Autodesk Fusion 360 part; units mm, degrees
note: some values were not read from the file. Chosen so that the rebuilt part matches the saved one: which face or edge a step refers to. Set by a fixed rule: which sketch regions a step uses.
(part 2 of 3)
  line L673 (81.1779, -7.0016) -> (84.5538, -8.9507)
  line L674 (81.1779, -3.1036) -> (81.1779, -7.0016)
  line L675 (84.5538, -1.1545) -> (81.1779, -3.1036)
  line L676 (87.9296, -3.1036) -> (84.5538, -1.1545)
  line L677 (84.5538, -8.9507) -> (87.9296, -7.0016)
  line L678 (83.9508, -13.893) -> (83.9508, -9.995)
  line L679 (83.9508, -9.995) -> (80.575, -8.0459)
  line L680 (80.575, -8.0459) -> (77.1992, -9.995)
  line L681 (77.1992, -9.995) -> (77.1992, -13.893)
  line L682 (77.1992, -13.893) -> (80.575, -15.8421)
  line L683 (80.575, -15.8421) -> (83.9508, -13.893)
  line L684 (87.9296, -7.0016) -> (87.9296, -3.1036)
  line L685 (9.5604, 6.9424) -> (12.9363, 4.9933)
  line L686 (9.5604, 10.8404) -> (9.5604, 6.9424)
  line L687 (12.9363, 12.7895) -> (9.5604, 10.8404)
  line L688 (16.3121, 10.8404) -> (12.9363, 12.7895)
  line L689 (12.9363, 4.9933) -> (16.3121, 6.9424)
  line L690 (12.3333, 0.051) -> (12.3333, 3.949)
  line L691 (12.3333, 3.949) -> (8.9575, 5.8981)
  line L692 (8.9575, 5.8981) -> (5.5817, 3.949)
  line L693 (5.5817, 3.949) -> (5.5817, 0.051)
  line L694 (5.5817, 0.051) -> (8.9575, -1.8981)
  line L695 (8.9575, -1.8981) -> (12.3333, 0.051)
  line L696 (16.3121, 6.9424) -> (16.3121, 10.8404)
  line L697 (17.5179, 6.9424) -> (20.8938, 4.9933)
  line L698 (17.5179, 10.8404) -> (17.5179, 6.9424)
  line L699 (20.8938, 12.7895) -> (17.5179, 10.8404)
  line L700 (24.2696, 10.8404) -> (20.8938, 12.7895)
  line L701 (20.8938, 4.9933) -> (24.2696, 6.9424)
  line L702 (20.2908, 0.051) -> (20.2908, 3.949)
  line L703 (20.2908, 3.949) -> (16.915, 5.8981)
  line L704 (16.915, 5.8981) -> (13.5392, 3.949)
  line L705 (13.5392, 3.949) -> (13.5392, 0.051)
  line L706 (13.5392, 0.051) -> (16.915, -1.8981)
  line L707 (16.915, -1.8981) -> (20.2908, 0.051)
  line L708 (24.2696, 6.9424) -> (24.2696, 10.8404)
  line L709 (25.4754, 6.9424) -> (28.8513, 4.9933)
  line L710 (25.4754, 10.8404) -> (25.4754, 6.9424)
  line L711 (28.8513, 12.7895) -> (25.4754, 10.8404)
  line L712 (32.2271, 10.8404) -> (28.8513, 12.7895)
  line L713 (28.8513, 4.9933) -> (32.2271, 6.9424)
  line L714 (28.2483, 0.051) -> (28.2483, 3.949)
  line L715 (28.2483, 3.949) -> (24.8725, 5.8981)
  line L716 (24.8725, 5.8981) -> (21.4967, 3.949)
  line L717 (21.4967, 3.949) -> (21.4967, 0.051)
  line L718 (21.4967, 0.051) -> (24.8725, -1.8981)
  line L719 (24.8725, -1.8981) -> (28.2483, 0.051)
  line L720 (32.2271, 6.9424) -> (32.2271, 10.8404)
  line L721 (33.4329, 6.9424) -> (36.8088, 4.9933)
  line L722 (33.4329, 10.8404) -> (33.4329, 6.9424)
  line L723 (36.8088, 12.7895) -> (33.4329, 10.8404)
  line L724 (40.1846, 10.8404) -> (36.8088, 12.7895)
  line L725 (36.8088, 4.9933) -> (40.1846, 6.9424)
  line L726 (36.2058, 0.051) -> (36.2058, 3.949)
  line L727 (36.2058, 3.949) -> (32.83, 5.8981)
  line L728 (32.83, 5.8981) -> (29.4542, 3.949)
  line L729 (29.4542, 3.949) -> (29.4542, 0.051)
  line L730 (29.4542, 0.051) -> (32.83, -1.8981)
  line L731 (32.83, -1.8981) -> (36.2058, 0.051)
  line L732 (40.1846, 6.9424) -> (40.1846, 10.8404)
  line L733 (41.3904, 6.9424) -> (44.7663, 4.9933)
  line L734 (41.3904, 10.8404) -> (41.3904, 6.9424)
  line L735 (44.7663, 12.7895) -> (41.3904, 10.8404)
  line L736 (48.1421, 10.8404) -> (44.7663, 12.7895)
  line L737 (44.7663, 4.9933) -> (48.1421, 6.9424)
  line L738 (44.1633, 0.051) -> (44.1633, 3.949)
  line L739 (44.1633, 3.949) -> (40.7875, 5.8981)
  line L740 (40.7875, 5.8981) -> (37.4117, 3.949)
  line L741 (37.4117, 3.949) -> (37.4117, 0.051)
  line L742 (37.4117, 0.051) -> (40.7875, -1.8981)
  line L743 (40.7875, -1.8981) -> (44.1633, 0.051)
  line L744 (48.1421, 6.9424) -> (48.1421, 10.8404)
  line L745 (49.3479, 6.9424) -> (52.7238, 4.9933)
  line L746 (49.3479, 10.8404) -> (49.3479, 6.9424)
  line L747 (52.7238, 12.7895) -> (49.3479, 10.8404)
  line L748 (56.0996, 10.8404) -> (52.7238, 12.7895)
  line L749 (52.7238, 4.9933) -> (56.0996, 6.9424)
  line L750 (52.1208, 0.051) -> (52.1208, 3.949)
  line L751 (52.1208, 3.949) -> (48.745, 5.8981)
  line L752 (48.745, 5.8981) -> (45.3692, 3.949)
  line L753 (45.3692, 3.949) -> (45.3692, 0.051)
  line L754 (45.3692, 0.051) -> (48.745, -1.8981)
  line L755 (48.745, -1.8981) -> (52.1208, 0.051)
  line L756 (56.0996, 6.9424) -> (56.0996, 10.8404)
  line L757 (57.3054, 6.9424) -> (60.6813, 4.9933)
  line L758 (57.3054, 10.8404) -> (57.3054, 6.9424)
  line L759 (60.6813, 12.7895) -> (57.3054, 10.8404)
  line L760 (64.0571, 10.8404) -> (60.6813, 12.7895)
  line L761 (60.6813, 4.9933) -> (64.0571, 6.9424)
  line L762 (60.0783, 0.051) -> (60.0783, 3.949)
  line L763 (60.0783, 3.949) -> (56.7025, 5.8981)
  line L764 (56.7025, 5.8981) -> (53.3267, 3.949)
  line L765 (53.3267, 3.949) -> (53.3267, 0.051)
  line L766 (53.3267, 0.051) -> (56.7025, -1.8981)
  line L767 (56.7025, -1.8981) -> (60.0783, 0.051)
  line L768 (64.0571, 6.9424) -> (64.0571, 10.8404)
  line L769 (65.2629, 6.9424) -> (68.6388, 4.9933)
  line L770 (65.2629, 10.8404) -> (65.2629, 6.9424)
  line L771 (68.6388, 12.7895) -> (65.2629, 10.8404)
  line L772 (72.0146, 10.8404) -> (68.6388, 12.7895)
  line L773 (68.6388, 4.9933) -> (72.0146, 6.9424)
  line L774 (68.0358, 0.051) -> (68.0358, 3.949)
  line L775 (68.0358, 3.949) -> (64.66, 5.8981)
  line L776 (64.66, 5.8981) -> (61.2842, 3.949)
  line L777 (61.2842, 3.949) -> (61.2842, 0.051)
  line L778 (61.2842, 0.051) -> (64.66, -1.8981)
  line L779 (64.66, -1.8981) -> (68.0358, 0.051)
  line L780 (72.0146, 6.9424) -> (72.0146, 10.8404)
  line L781 (73.2204, 6.9424) -> (76.5963, 4.9933)
  line L782 (73.2204, 10.8404) -> (73.2204, 6.9424)
  line L783 (76.5963, 12.7895) -> (73.2204, 10.8404)
  line L784 (79.9721, 10.8404) -> (76.5963, 12.7895)
  line L785 (76.5963, 4.9933) -> (79.9721, 6.9424)
  line L786 (75.9933, 0.051) -> (75.9933, 3.949)
  line L787 (75.9933, 3.949) -> (72.6175, 5.8981)
  line L788 (72.6175, 5.8981) -> (69.2417, 3.949)
  line L789 (69.2417, 3.949) -> (69.2417, 0.051)
  line L790 (69.2417, 0.051) -> (72.6175, -1.8981)
  line L791 (72.6175, -1.8981) -> (75.9933, 0.051)
  line L792 (79.9721, 6.9424) -> (79.9721, 10.8404)
  line L793 (81.1779, 6.9424) -> (84.5538, 4.9933)
  line L794 (81.1779, 10.8404) -> (81.1779, 6.9424)
  line L795 (84.5538, 12.7895) -> (81.1779, 10.8404)
  line L796 (87.9296, 10.8404) -> (84.5538, 12.7895)
  line L797 (84.5538, 4.9933) -> (87.9296, 6.9424)
  line L798 (83.9508, 0.051) -> (83.9508, 3.949)
  line L799 (83.9508, 3.949) -> (80.575, 5.8981)
  line L800 (80.575, 5.8981) -> (77.1992, 3.949)
  line L801 (77.1992, 3.949) -> (77.1992, 0.051)
  line L802 (77.1992, 0.051) -> (80.575, -1.8981)
  line L803 (80.575, -1.8981) -> (83.9508, 0.051)
  line L804 (87.9296, 6.9424) -> (87.9296, 10.8404)
  line L805 (1.6029, 20.8864) -> (4.9788, 18.9373)
  line L806 (1.6029, 24.7844) -> (1.6029, 20.8864)
  line L807 (4.9788, 26.7335) -> (1.6029, 24.7844)
  line L808 (8.3546, 24.7844) -> (4.9788, 26.7335)
  line L809 (4.9788, 18.9373) -> (8.3546, 20.8864)
  line L810 (4.3758, 13.995) -> (4.3758, 17.893)
  line L811 (4.3758, 17.893) -> (1, 19.8421)
  line L812 (1, 19.8421) -> (-2.3758, 17.893)
  line L813 (-2.3758, 17.893) -> (-2.3758, 13.995)
  line L814 (-2.3758, 13.995) -> (1, 12.0459)
  line L815 (1, 12.0459) -> (4.3758, 13.995)
  line L816 (8.3546, 20.8864) -> (8.3546, 24.7844)
  line L817 (9.5604, 20.8864) -> (12.9363, 18.9373)
  line L818 (9.5604, 24.7844) -> (9.5604, 20.8864)
  line L819 (12.9363, 26.7335) -> (9.5604, 24.7844)
  line L820 (16.3121, 24.7844) -> (12.9363, 26.7335)
  line L821 (12.9363, 18.9373) -> (16.3121, 20.8864)
  line L822 (12.3333, 13.995) -> (12.3333, 17.893)
  line L823 (12.3333, 17.893) -> (8.9575, 19.8421)
  line L824 (8.9575, 19.8421) -> (5.5817, 17.893)
  line L825 (5.5817, 17.893) -> (5.5817, 13.995)
  line L826 (5.5817, 13.995) -> (8.9575, 12.0459)
  line L827 (8.9575, 12.0459) -> (12.3333, 13.995)
  line L828 (16.3121, 20.8864) -> (16.3121, 24.7844)
  line L829 (17.5179, 20.8864) -> (20.8938, 18.9373)
  line L830 (17.5179, 24.7844) -> (17.5179, 20.8864)
  line L831 (20.8938, 26.7335) -> (17.5179, 24.7844)
  line L832 (24.2696, 24.7844) -> (20.8938, 26.7335)
  line L833 (20.8938, 18.9373) -> (24.2696, 20.8864)
  line L834 (20.2908, 13.995) -> (20.2908, 17.893)
  line L835 (20.2908, 17.893) -> (16.915, 19.8421)
  line L836 (16.915, 19.8421) -> (13.5392, 17.893)
  line L837 (13.5392, 17.893) -> (13.5392, 13.995)
  line L838 (13.5392, 13.995) -> (16.915, 12.0459)
  line L839 (16.915, 12.0459) -> (20.2908, 13.995)
  line L840 (24.2696, 20.8864) -> (24.2696, 24.7844)
  line L841 (25.4754, 20.8864) -> (28.8513, 18.9373)
  line L842 (25.4754, 24.7844) -> (25.4754, 20.8864)
  line L843 (28.8513, 26.7335) -> (25.4754, 24.7844)
  line L844 (32.2271, 24.7844) -> (28.8513, 26.7335)
  line L845 (28.8513, 18.9373) -> (32.2271, 20.8864)
  line L846 (28.2483, 13.995) -> (28.2483, 17.893)
  line L847 (28.2483, 17.893) -> (24.8725, 19.8421)
  line L848 (24.8725, 19.8421) -> (21.4967, 17.893)
  line L849 (21.4967, 17.893) -> (21.4967, 13.995)
  line L850 (21.4967, 13.995) -> (24.8725, 12.0459)
  line L851 (24.8725, 12.0459) -> (28.2483, 13.995)
  line L852 (32.2271, 20.8864) -> (32.2271, 24.7844)
  line L853 (33.4329, 20.8864) -> (36.8088, 18.9373)
  line L854 (33.4329, 24.7844) -> (33.4329, 20.8864)
  line L855 (36.8088, 26.7335) -> (33.4329, 24.7844)
  line L856 (40.1846, 24.7844) -> (36.8088, 26.7335)
  line L857 (36.8088, 18.9373) -> (40.1846, 20.8864)
  line L858 (36.2058, 13.995) -> (36.2058, 17.893)
  line L859 (36.2058, 17.893) -> (32.83, 19.8421)
  line L860 (32.83, 19.8421) -> (29.4542, 17.893)
  line L861 (29.4542, 17.893) -> (29.4542, 13.995)
  line L862 (29.4542, 13.995) -> (32.83, 12.0459)
  line L863 (32.83, 12.0459) -> (36.2058, 13.995)
  line L864 (40.1846, 20.8864) -> (40.1846, 24.7844)
  line L865 (41.3904, 20.8864) -> (44.7663, 18.9373)
  line L866 (41.3904, 24.7844) -> (41.3904, 20.8864)
  line L867 (44.7663, 26.7335) -> (41.3904, 24.7844)
  line L868 (48.1421, 24.7844) -> (44.7663, 26.7335)
  line L869 (44.7663, 18.9373) -> (48.1421, 20.8864)
  line L870 (44.1633, 13.995) -> (44.1633, 17.893)
  line L871 (44.1633, 17.893) -> (40.7875, 19.8421)
  line L872 (40.7875, 19.8421) -> (37.4117, 17.893)
  line L873 (37.4117, 17.893) -> (37.4117, 13.995)
  line L874 (37.4117, 13.995) -> (40.7875, 12.0459)
  line L875 (40.7875, 12.0459) -> (44.1633, 13.995)
  line L876 (48.1421, 20.8864) -> (48.1421, 24.7844)
  line L877 (49.3479, 20.8864) -> (52.7238, 18.9373)
  line L878 (49.3479, 24.7844) -> (49.3479, 20.8864)
  line L879 (52.7238, 26.7335) -> (49.3479, 24.7844)
  line L880 (56.0996, 24.7844) -> (52.7238, 26.7335)
  line L881 (52.7238, 18.9373) -> (56.0996, 20.8864)
  line L882 (52.1208, 13.995) -> (52.1208, 17.893)
  line L883 (52.1208, 17.893) -> (48.745, 19.8421)
  line L884 (48.745, 19.8421) -> (45.3692, 17.893)
  line L885 (45.3692, 17.893) -> (45.3692, 13.995)
  line L886 (45.3692, 13.995) -> (48.745, 12.0459)
  line L887 (48.745, 12.0459) -> (52.1208, 13.995)
  line L888 (56.0996, 20.8864) -> (56.0996, 24.7844)
  line L889 (57.3054, 20.8864) -> (60.6813, 18.9373)
  line L890 (57.3054, 24.7844) -> (57.3054, 20.8864)
  line L891 (60.6813, 26.7335) -> (57.3054, 24.7844)
  line L892 (64.0571, 24.7844) -> (60.6813, 26.7335)
  line L893 (60.6813, 18.9373) -> (64.0571, 20.8864)
  line L894 (60.0783, 13.995) -> (60.0783, 17.893)
  line L895 (60.0783, 17.893) -> (56.7025, 19.8421)
  line L896 (56.7025, 19.8421) -> (53.3267, 17.893)
  line L897 (53.3267, 17.893) -> (53.3267, 13.995)
  line L898 (53.3267, 13.995) -> (56.7025, 12.0459)
  line L899 (56.7025, 12.0459) -> (60.0783, 13.995)
  line L900 (64.0571, 20.8864) -> (64.0571, 24.7844)
  line L901 (65.2629, 20.8864) -> (68.6388, 18.9373)
  line L902 (65.2629, 24.7844) -> (65.2629, 20.8864)
  line L903 (68.6388, 26.7335) -> (65.2629, 24.7844)
  line L904 (72.0146, 24.7844) -> (68.6388, 26.7335)
  line L905 (68.6388, 18.9373) -> (72.0146, 20.8864)
  line L906 (68.0358, 13.995) -> (68.0358, 17.893)
  line L907 (68.0358, 17.893) -> (64.66, 19.8421)
  line L908 (64.66, 19.8421) -> (61.2842, 17.893)
  line L909 (61.2842, 17.893) -> (61.2842, 13.995)
  line L910 (61.2842, 13.995) -> (64.66, 12.0459)
  line L911 (64.66, 12.0459) -> (68.0358, 13.995)
  line L912 (72.0146, 20.8864) -> (72.0146, 24.7844)
  line L913 (73.2204, 20.8864) -> (76.5963, 18.9373)
  line L914 (73.2204, 24.7844) -> (73.2204, 20.8864)
  line L915 (76.5963, 26.7335) -> (73.2204, 24.7844)
  line L916 (79.9721, 24.7844) -> (76.5963, 26.7335)
  line L917 (76.5963, 18.9373) -> (79.9721, 20.8864)
  line L918 (75.9933, 13.995) -> (75.9933, 17.893)
  line L919 (75.9933, 17.893) -> (72.6175, 19.8421)
  line L920 (72.6175, 19.8421) -> (69.2417, 17.893)
  line L921 (69.2417, 17.893) -> (69.2417, 13.995)
  line L922 (69.2417, 13.995) -> (72.6175, 12.0459)
  line L923 (72.6175, 12.0459) -> (75.9933, 13.995)
  line L924 (79.9721, 20.8864) -> (79.9721, 24.7844)
  line L925 (81.1779, 20.8864) -> (84.5538, 18.9373)
  line L926 (81.1779, 24.7844) -> (81.1779, 20.8864)
  line L927 (84.5538, 26.7335) -> (81.1779, 24.7844)
  line L928 (87.9296, 24.7844) -> (84.5538, 26.7335)
  line L929 (84.5538, 18.9373) -> (87.9296, 20.8864)
  line L930 (83.9508, 13.995) -> (83.9508, 17.893)
  line L931 (83.9508, 17.893) -> (80.575, 19.8421)
  line L932 (80.575, 19.8421) -> (77.1992, 17.893)
  line L933 (77.1992, 17.893) -> (77.1992, 13.995)
  line L934 (77.1992, 13.995) -> (80.575, 12.0459)
  line L935 (80.575, 12.0459) -> (83.9508, 13.995)
  line L936 (87.9296, 20.8864) -> (87.9296, 24.7844)
  line L937 (1.6029, 34.8304) -> (4.9788, 32.8813)
  line L938 (1.6029, 38.7284) -> (1.6029, 34.8304)
  line L939 (4.9788, 40.6775) -> (1.6029, 38.7284)
  line L940 (8.3546, 38.7284) -> (4.9788, 40.6775)
  line L941 (4.9788, 32.8813) -> (8.3546, 34.8304)
  line L942 (4.3758, 27.939) -> (4.3758, 31.837)
  line L943 (4.3758, 31.837) -> (1, 33.7861)
  line L944 (1, 33.7861) -> (-2.3758, 31.837)
  line L945 (-2.3758, 31.837) -> (-2.3758, 27.939)
  line L946 (-2.3758, 27.939) -> (1, 25.9899)
  line L947 (1, 25.9899) -> (4.3758, 27.939)
  line L948 (8.3546, 34.8304) -> (8.3546, 38.7284)
  line L949 (9.5604, 34.8304) -> (12.9363, 32.8813)
  line L950 (9.5604, 38.7284) -> (9.5604, 34.8304)
  line L951 (12.9363, 40.6775) -> (9.5604, 38.7284)
  line L952 (16.3121, 38.7284) -> (12.9363, 40.6775)
  line L953 (12.9363, 32.8813) -> (16.3121, 34.8304)
  line L954 (12.3333, 27.939) -> (12.3333, 31.837)
  line L955 (12.3333, 31.837) -> (8.9575, 33.7861)
  line L956 (8.9575, 33.7861) -> (5.5817, 31.837)
  line L957 (5.5817, 31.837) -> (5.5817, 27.939)
  line L958 (5.5817, 27.939) -> (8.9575, 25.9899)
  line L959 (8.9575, 25.9899) -> (12.3333, 27.939)
  line L960 (16.3121, 34.8304) -> (16.3121, 38.7284)
  line L961 (17.5179, 34.8304) -> (20.8938, 32.8813)
  line L962 (17.5179, 38.7284) -> (17.5179, 34.8304)
  line L963 (20.8938, 40.6775) -> (17.5179, 38.7284)
  line L964 (24.2696, 38.7284) -> (20.8938, 40.6775)
  line L965 (20.8938, 32.8813) -> (24.2696, 34.8304)
  line L966 (20.2908, 27.939) -> (20.2908, 31.837)
  line L967 (20.2908, 31.837) -> (16.915, 33.7861)
  line L968 (16.915, 33.7861) -> (13.5392, 31.837)
  line L969 (13.5392, 31.837) -> (13.5392, 27.939)
  line L970 (13.5392, 27.939) -> (16.915, 25.9899)
  line L971 (16.915, 25.9899) -> (20.2908, 27.939)
  line L972 (24.2696, 34.8304) -> (24.2696, 38.7284)
  line L973 (25.4754, 34.8304) -> (28.8513, 32.8813)
  line L974 (25.4754, 38.7284) -> (25.4754, 34.8304)
  line L975 (28.8513, 40.6775) -> (25.4754, 38.7284)
  line L976 (32.2271, 38.7284) -> (28.8513, 40.6775)
  line L977 (28.8513, 32.8813) -> (32.2271, 34.8304)
  line L978 (28.2483, 27.939) -> (28.2483, 31.837)
  line L979 (28.2483, 31.837) -> (24.8725, 33.7861)
  line L980 (24.8725, 33.7861) -> (21.4967, 31.837)
  line L981 (21.4967, 31.837) -> (21.4967, 27.939)
  line L982 (21.4967, 27.939) -> (24.8725, 25.9899)
  line L983 (24.8725, 25.9899) -> (28.2483, 27.939)
  line L984 (32.2271, 34.8304) -> (32.2271, 38.7284)
  line L985 (33.4329, 34.8304) -> (36.8088, 32.8813)
  line L986 (33.4329, 38.7284) -> (33.4329, 34.8304)
  line L987 (36.8088, 40.6775) -> (33.4329, 38.7284)
  line L988 (40.1846, 38.7284) -> (36.8088, 40.6775)
  line L989 (36.8088, 32.8813) -> (40.1846, 34.8304)
  line L990 (36.2058, 27.939) -> (36.2058, 31.837)
  line L991 (36.2058, 31.837) -> (32.83, 33.7861)
  line L992 (32.83, 33.7861) -> (29.4542, 31.837)
  line L993 (29.4542, 31.837) -> (29.4542, 27.939)
  line L994 (29.4542, 27.939) -> (32.83, 25.9899)
  line L995 (32.83, 25.9899) -> (36.2058, 27.939)
  line L996 (40.1846, 34.8304) -> (40.1846, 38.7284)
  line L997 (41.3904, 34.8304) -> (44.7663, 32.8813)
  line L998 (41.3904, 38.7284) -> (41.3904, 34.8304)
  line L999 (44.7663, 40.6775) -> (41.3904, 38.7284)
  line L1000 (48.1421, 38.7284) -> (44.7663, 40.6775)
  line L1001 (44.7663, 32.8813) -> (48.1421, 34.8304)
  line L1002 (44.1633, 27.939) -> (44.1633, 31.837)
  line L1003 (44.1633, 31.837) -> (40.7875, 33.7861)
  line L1004 (40.7875, 33.7861) -> (37.4117, 31.837)
  line L1005 (37.4117, 31.837) -> (37.4117, 27.939)
  line L1006 (37.4117, 27.939) -> (40.7875, 25.9899)
  line L1007 (40.7875, 25.9899) -> (44.1633, 27.939)
  line L1008 (48.1421, 34.8304) -> (48.1421, 38.7284)
  line L1009 (49.3479, 34.8304) -> (52.7238, 32.8813)
  line L1010 (49.3479, 38.7284) -> (49.3479, 34.8304)
  line L1011 (52.7238, 40.6775) -> (49.3479, 38.7284)
  line L1012 (56.0996, 38.7284) -> (52.7238, 40.6775)
  line L1013 (52.7238, 32.8813) -> (56.0996, 34.8304)
  line L1014 (52.1208, 27.939) -> (52.1208, 31.837)
  line L1015 (52.1208, 31.837) -> (48.745, 33.7861)
  line L1016 (48.745, 33.7861) -> (45.3692, 31.837)
  line L1017 (45.3692, 31.837) -> (45.3692, 27.939)
  line L1018 (45.3692, 27.939) -> (48.745, 25.9899)
  line L1019 (48.745, 25.9899) -> (52.1208, 27.939)
  line L1020 (56.0996, 34.8304) -> (56.0996, 38.7284)
  line L1021 (57.3054, 34.8304) -> (60.6813, 32.8813)
  line L1022 (57.3054, 38.7284) -> (57.3054, 34.8304)
  line L1023 (60.6813, 40.6775) -> (57.3054, 38.7284)
  line L1024 (64.0571, 38.7284) -> (60.6813, 40.6775)
  line L1025 (60.6813, 32.8813) -> (64.0571, 34.8304)
  line L1026 (60.0783, 27.939) -> (60.0783, 31.837)
  line L1027 (60.0783, 31.837) -> (56.7025, 33.7861)
  line L1028 (56.7025, 33.7861) -> (53.3267, 31.837)
  line L1029 (53.3267, 31.837) -> (53.3267, 27.939)
  line L1030 (53.3267, 27.939) -> (56.7025, 25.9899)
  line L1031 (56.7025, 25.9899) -> (60.0783, 27.939)
  line L1032 (64.0571, 34.8304) -> (64.0571, 38.7284)
  line L1033 (65.2629, 34.8304) -> (68.6388, 32.8813)
  line L1034 (65.2629, 38.7284) -> (65.2629, 34.8304)
  line L1035 (68.6388, 40.6775) -> (65.2629, 38.7284)
  line L1036 (72.0146, 38.7284) -> (68.6388, 40.6775)
  line L1037 (68.6388, 32.8813) -> (72.0146, 34.8304)
  line L1038 (68.0358, 27.939) -> (68.0358, 31.837)
  line L1039 (68.0358, 31.837) -> (64.66, 33.7861)
  line L1040 (64.66, 33.7861) -> (61.2842, 31.837)
  line L1041 (61.2842, 31.837) -> (61.2842, 27.939)
  line L1042 (61.2842, 27.939) -> (64.66, 25.9899)
  line L1043 (64.66, 25.9899) -> (68.0358, 27.939)
  line L1044 (72.0146, 34.8304) -> (72.0146, 38.7284)
  line L1045 (73.2204, 34.8304) -> (76.5963, 32.8813)
  line L1046 (73.2204, 38.7284) -> (73.2204, 34.8304)
  line L1047 (76.5963, 40.6775) -> (73.2204, 38.7284)
  line L1048 (79.9721, 38.7284) -> (76.5963, 40.6775)
  line L1049 (76.5963, 32.8813) -> (79.9721, 34.8304)
  line L1050 (75.9933, 27.939) -> (75.9933, 31.837)
  line L1051 (75.9933, 31.837) -> (72.6175, 33.7861)
  line L1052 (72.6175, 33.7861) -> (69.2417, 31.837)
  line L1053 (69.2417, 31.837) -> (69.2417, 27.939)
  line L1054 (69.2417, 27.939) -> (72.6175, 25.9899)
  line L1055 (72.6175, 25.9899) -> (75.9933, 27.939)
  line L1056 (79.9721, 34.8304) -> (79.9721, 38.7284)
  line L1057 (81.1779, 34.8304) -> (84.5538, 32.8813)
  line L1058 (81.1779, 38.7284) -> (81.1779, 34.8304)
  line L1059 (84.5538, 40.6775) -> (81.1779, 38.7284)
  line L1060 (87.9296, 38.7284) -> (84.5538, 40.6775)
  line L1061 (84.5538, 32.8813) -> (87.9296, 34.8304)
  line L1062 (83.9508, 27.939) -> (83.9508, 31.837)
  line L1063 (83.9508, 31.837) -> (80.575, 33.7861)
  line L1064 (80.575, 33.7861) -> (77.1992, 31.837)
  line L1065 (77.1992, 31.837) -> (77.1992, 27.939)
  line L1066 (77.1992, 27.939) -> (80.575, 25.9899)
  line L1067 (80.575, 25.9899) -> (83.9508, 27.939)
  line L1068 (87.9296, 34.8304) -> (87.9296, 38.7284)
  line L1069 (1.6029, 48.7744) -> (4.9788, 46.8253)
  line L1070 (1.6029, 52.6724) -> (1.6029, 48.7744)
  line L1071 (4.9788, 54.6215) -> (1.6029, 52.6724)
  line L1072 (8.3546, 52.6724) -> (4.9788, 54.6215)
  line L1073 (4.9788, 46.8253) -> (8.3546, 48.7744)
  line L1074 (4.3758, 41.883) -> (4.3758, 45.781)
  line L1075 (4.3758, 45.781) -> (1, 47.7301)
  line L1076 (1, 47.7301) -> (-2.3758, 45.781)
  line L1077 (-2.3758, 45.781) -> (-2.3758, 41.883)
  line L1078 (-2.3758, 41.883) -> (1, 39.9339)
  line L1079 (1, 39.9339) -> (4.3758, 41.883)
  line L1080 (8.3546, 48.7744) -> (8.3546, 52.6724)
  line L1081 (9.5604, 48.7744) -> (12.9363, 46.8253)
  line L1082 (9.5604, 52.6724) -> (9.5604, 48.7744)
  line L1083 (12.9363, 54.6215) -> (9.5604, 52.6724)
  line L1084 (16.3121, 52.6724) -> (12.9363, 54.6215)
  line L1085 (12.9363, 46.8253) -> (16.3121, 48.7744)
  line L1086 (12.3333, 41.883) -> (12.3333, 45.781)
  line L1087 (12.3333, 45.781) -> (8.9575, 47.7301)
  line L1088 (8.9575, 47.7301) -> (5.5817, 45.781)
  line L1089 (5.5817, 45.781) -> (5.5817, 41.883)
  line L1090 (5.5817, 41.883) -> (8.9575, 39.9339)
  line L1091 (8.9575, 39.9339) -> (12.3333, 41.883)
  line L1092 (16.3121, 48.7744) -> (16.3121, 52.6724)
  line L1093 (17.5179, 48.7744) -> (20.8938, 46.8253)
  line L1094 (17.5179, 52.6724) -> (17.5179, 48.7744)
  line L1095 (20.8938, 54.6215) -> (17.5179, 52.6724)
  line L1096 (24.2696, 52.6724) -> (20.8938, 54.6215)
  line L1097 (20.8938, 46.8253) -> (24.2696, 48.7744)
  line L1098 (20.2908, 41.883) -> (20.2908, 45.781)
  line L1099 (20.2908, 45.781) -> (16.915, 47.7301)
  line L1100 (16.915, 47.7301) -> (13.5392, 45.781)
  line L1101 (13.5392, 45.781) -> (13.5392, 41.883)
  line L1102 (13.5392, 41.883) -> (16.915, 39.9339)
  line L1103 (16.915, 39.9339) -> (20.2908, 41.883)
  line L1104 (24.2696, 48.7744) -> (24.2696, 52.6724)
  line L1105 (25.4754, 48.7744) -> (28.8513, 46.8253)
  line L1106 (25.4754, 52.6724) -> (25.4754, 48.7744)
  line L1107 (28.8513, 54.6215) -> (25.4754, 52.6724)
  line L1108 (32.2271, 52.6724) -> (28.8513, 54.6215)
  line L1109 (28.8513, 46.8253) -> (32.2271, 48.7744)
  line L1110 (28.2483, 41.883) -> (28.2483, 45.781)
  line L1111 (28.2483, 45.781) -> (24.8725, 47.7301)
  line L1112 (24.8725, 47.7301) -> (21.4967, 45.781)
  line L1113 (21.4967, 45.781) -> (21.4967, 41.883)
  line L1114 (21.4967, 41.883) -> (24.8725, 39.9339)
  line L1115 (24.8725, 39.9339) -> (28.2483, 41.883)
  line L1116 (32.2271, 48.7744) -> (32.2271, 52.6724)
  line L1117 (33.4329, 48.7744) -> (36.8088, 46.8253)
  line L1118 (33.4329, 52.6724) -> (33.4329, 48.7744)
  line L1119 (36.8088, 54.6215) -> (33.4329, 52.6724)
  line L1120 (40.1846, 52.6724) -> (36.8088, 54.6215)
  line L1121 (36.8088, 46.8253) -> (40.1846, 48.7744)
  line L1122 (36.2058, 41.883) -> (36.2058, 45.781)
  line L1123 (36.2058, 45.781) -> (32.83, 47.7301)
  line L1124 (32.83, 47.7301) -> (29.4542, 45.781)
  line L1125 (29.4542, 45.781) -> (29.4542, 41.883)
  line L1126 (29.4542, 41.883) -> (32.83, 39.9339)
  line L1127 (32.83, 39.9339) -> (36.2058, 41.883)
  line L1128 (40.1846, 48.7744) -> (40.1846, 52.6724)
  line L1129 (41.3904, 48.7744) -> (44.7663, 46.8253)
  line L1130 (41.3904, 52.6724) -> (41.3904, 48.7744)
  line L1131 (44.7663, 54.6215) -> (41.3904, 52.6724)
  line L1132 (48.1421, 52.6724) -> (44.7663, 54.6215)
  line L1133 (44.7663, 46.8253) -> (48.1421, 48.7744)
  line L1134 (44.1633, 41.883) -> (44.1633, 45.781)
  line L1135 (44.1633, 45.781) -> (40.7875, 47.7301)
  line L1136 (40.7875, 47.7301) -> (37.4117, 45.781)
  line L1137 (37.4117, 45.781) -> (37.4117, 41.883)
  line L1138 (37.4117, 41.883) -> (40.7875, 39.9339)
  line L1139 (40.7875, 39.9339) -> (44.1633, 41.883)
  line L1140 (48.1421, 48.7744) -> (48.1421, 52.6724)
  line L1141 (49.3479, 48.7744) -> (52.7238, 46.8253)
  line L1142 (49.3479, 52.6724) -> (49.3479, 48.7744)
  line L1143 (52.7238, 54.6215) -> (49.3479, 52.6724)
  line L1144 (56.0996, 52.6724) -> (52.7238, 54.6215)
  line L1145 (52.7238, 46.8253) -> (56.0996, 48.7744)
  line L1146 (52.1208, 41.883) -> (52.1208, 45.781)
  line L1147 (52.1208, 45.781) -> (48.745, 47.7301)
  line L1148 (48.745, 47.7301) -> (45.3692, 45.781)
  line L1149 (45.3692, 45.781) -> (45.3692, 41.883)
  line L1150 (45.3692, 41.883) -> (48.745, 39.9339)
  line L1151 (48.745, 39.9339) -> (52.1208, 41.883)
  line L1152 (56.0996, 48.7744) -> (56.0996, 52.6724)
  line L1153 (57.3054, 48.7744) -> (60.6813, 46.8253)
  line L1154 (57.3054, 52.6724) -> (57.3054, 48.7744)
  line L1155 (60.6813, 54.6215) -> (57.3054, 52.6724)
  line L1156 (64.0571, 52.6724) -> (60.6813, 54.6215)
  line L1157 (60.6813, 46.8253) -> (64.0571, 48.7744)
  line L1158 (60.0783, 41.883) -> (60.0783, 45.781)
  line L1159 (60.0783, 45.781) -> (56.7025, 47.7301)
  line L1160 (56.7025, 47.7301) -> (53.3267, 45.781)
  line L1161 (53.3267, 45.781) -> (53.3267, 41.883)
  line L1162 (53.3267, 41.883) -> (56.7025, 39.9339)
  line L1163 (56.7025, 39.9339) -> (60.0783, 41.883)
  line L1164 (64.0571, 48.7744) -> (64.0571, 52.6724)
  line L1165 (65.2629, 48.7744) -> (68.6388, 46.8253)
  line L1166 (65.2629, 52.6724) -> (65.2629, 48.7744)
  line L1167 (68.6388, 54.6215) -> (65.2629, 52.6724)
  line L1168 (72.0146, 52.6724) -> (68.6388, 54.6215)
  line L1169 (68.6388, 46.8253) -> (72.0146, 48.7744)
  line L1170 (68.0358, 41.883) -> (68.0358, 45.781)
  line L1171 (68.0358, 45.781) -> (64.66, 47.7301)
  line L1172 (64.66, 47.7301) -> (61.2842, 45.781)
  line L1173 (61.2842, 45.781) -> (61.2842, 41.883)
  line L1174 (61.2842, 41.883) -> (64.66, 39.9339)
  line L1175 (64.66, 39.9339) -> (68.0358, 41.883)
  line L1176 (72.0146, 48.7744) -> (72.0146, 52.6724)
  line L1177 (73.2204, 48.7744) -> (76.5963, 46.8253)
  line L1178 (73.2204, 52.6724) -> (73.2204, 48.7744)
  line L1179 (76.5963, 54.6215) -> (73.2204, 52.6724)
  line L1180 (79.9721, 52.6724) -> (76.5963, 54.6215)
  line L1181 (76.5963, 46.8253) -> (79.9721, 48.7744)
  line L1182 (75.9933, 41.883) -> (75.9933, 45.781)
  line L1183 (75.9933, 45.781) -> (72.6175, 47.7301)
  line L1184 (72.6175, 47.7301) -> (69.2417, 45.781)
  line L1185 (69.2417, 45.781) -> (69.2417, 41.883)
  line L1186 (69.2417, 41.883) -> (72.6175, 39.9339)
  line L1187 (72.6175, 39.9339) -> (75.9933, 41.883)
  line L1188 (79.9721, 48.7744) -> (79.9721, 52.6724)
  line L1189 (81.1779, 48.7744) -> (84.5538, 46.8253)
  line L1190 (81.1779, 52.6724) -> (81.1779, 48.7744)
  line L1191 (84.5538, 54.6215) -> (81.1779, 52.6724)
  line L1192 (87.9296, 52.6724) -> (84.5538, 54.6215)
  line L1193 (84.5538, 46.8253) -> (87.9296, 48.7744)
  line L1194 (83.9508, 41.883) -> (83.9508, 45.781)
  line L1195 (83.9508, 45.781) -> (80.575, 47.7301)
  line L1196 (80.575, 47.7301) -> (77.1992, 45.781)
  line L1197 (77.1992, 45.781) -> (77.1992, 41.883)
  line L1198 (77.1992, 41.883) -> (80.575, 39.9339)
  line L1199 (80.575, 39.9339) -> (83.9508, 41.883)
  line L1200 (87.9296, 48.7744) -> (87.9296, 52.6724)
  line L1201 (1.6029, 62.7184) -> (4.9788, 60.7693)
  line L1202 (1.6029, 66.6164) -> (1.6029, 62.7184)
  line L1203 (4.9788, 68.5655) -> (1.6029, 66.6164)
  line L1204 (8.3546, 66.6164) -> (4.9788, 68.5655)
  line L1205 (4.9788, 60.7693) -> (8.3546, 62.7184)
  line L1206 (4.3758, 55.827) -> (4.3758, 59.725)
  line L1207 (4.3758, 59.725) -> (1, 61.6741)
  line L1208 (1, 61.6741) -> (-2.3758, 59.725)
  line L1209 (-2.3758, 59.725) -> (-2.3758, 55.827)
  line L1210 (-2.3758, 55.827) -> (1, 53.8779)
  line L1211 (1, 53.8779) -> (4.3758, 55.827)
  line L1212 (8.3546, 62.7184) -> (8.3546, 66.6164)
  line L1213 (9.5604, 62.7184) -> (12.9363, 60.7693)
  line L1214 (9.5604, 66.6164) -> (9.5604, 62.7184)
  line L1215 (12.9363, 68.5655) -> (9.5604, 66.6164)
  line L1216 (16.3121, 66.6164) -> (12.9363, 68.5655)
  line L1217 (12.9363, 60.7693) -> (16.3121, 62.7184)
  line L1218 (12.3333, 55.827) -> (12.3333, 59.725)
  line L1219 (12.3333, 59.725) -> (8.9575, 61.6741)
  line L1220 (8.9575, 61.6741) -> (5.5817, 59.725)
  line L1221 (5.5817, 59.725) -> (5.5817, 55.827)
  line L1222 (5.5817, 55.827) -> (8.9575, 53.8779)
  line L1223 (8.9575, 53.8779) -> (12.3333, 55.827)
  line L1224 (16.3121, 62.7184) -> (16.3121, 66.6164)
  line L1225 (17.5179, 62.7184) -> (20.8938, 60.7693)
  line L1226 (17.5179, 66.6164) -> (17.5179, 62.7184)
  line L1227 (20.8938, 68.5655) -> (17.5179, 66.6164)
  line L1228 (24.2696, 66.6164) -> (20.8938, 68.5655)
  line L1229 (20.8938, 60.7693) -> (24.2696, 62.7184)
  line L1230 (20.2908, 55.827) -> (20.2908, 59.725)
  line L1231 (20.2908, 59.725) -> (16.915, 61.6741)
  line L1232 (16.915, 61.6741) -> (13.5392, 59.725)
  line L1233 (13.5392, 59.725) -> (13.5392, 55.827)
  line L1234 (13.5392, 55.827) -> (16.915, 53.8779)
  line L1235 (16.915, 53.8779) -> (20.2908, 55.827)
  line L1236 (24.2696, 62.7184) -> (24.2696, 66.6164)
  line L1237 (25.4754, 62.7184) -> (28.8513, 60.7693)
  line L1238 (25.4754, 66.6164) -> (25.4754, 62.7184)
  line L1239 (28.8513, 68.5655) -> (25.4754, 66.6164)
  line L1240 (32.2271, 66.6164) -> (28.8513, 68.5655)
  line L1241 (28.8513, 60.7693) -> (32.2271, 62.7184)
  line L1242 (28.2483, 55.827) -> (28.2483, 59.725)
  line L1243 (28.2483, 59.725) -> (24.8725, 61.6741)
  line L1244 (24.8725, 61.6741) -> (21.4967, 59.725)
  line L1245 (21.4967, 59.725) -> (21.4967, 55.827)
  line L1246 (21.4967, 55.827) -> (24.8725, 53.8779)
  line L1247 (24.8725, 53.8779) -> (28.2483, 55.827)
  line L1248 (32.2271, 62.7184) -> (32.2271, 66.6164)
  line L1249 (33.4329, 62.7184) -> (36.8088, 60.7693)
  line L1250 (33.4329, 66.6164) -> (33.4329, 62.7184)
  line L1251 (36.8088, 68.5655) -> (33.4329, 66.6164)
  line L1252 (40.1846, 66.6164) -> (36.8088, 68.5655)
  line L1253 (36.8088, 60.7693) -> (40.1846, 62.7184)
  line L1254 (36.2058, 55.827) -> (36.2058, 59.725)
  line L1255 (36.2058, 59.725) -> (32.83, 61.6741)
  line L1256 (32.83, 61.6741) -> (29.4542, 59.725)
  line L1257 (29.4542, 59.725) -> (29.4542, 55.827)
  line L1258 (29.4542, 55.827) -> (32.83, 53.8779)
  line L1259 (32.83, 53.8779) -> (36.2058, 55.827)
  line L1260 (40.1846, 62.7184) -> (40.1846, 66.6164)
  line L1261 (41.3904, 62.7184) -> (44.7663, 60.7693)
  line L1262 (41.3904, 66.6164) -> (41.3904, 62.7184)
  line L1263 (44.7663, 68.5655) -> (41.3904, 66.6164)
  line L1264 (48.1421, 66.6164) -> (44.7663, 68.5655)
  line L1265 (44.7663, 60.7693) -> (48.1421, 62.7184)
  line L1266 (44.1633, 55.827) -> (44.1633, 59.725)
  line L1267 (44.1633, 59.725) -> (40.7875, 61.6741)
  line L1268 (40.7875, 61.6741) -> (37.4117, 59.725)
  line L1269 (37.4117, 59.725) -> (37.4117, 55.827)
  line L1270 (37.4117, 55.827) -> (40.7875, 53.8779)
  line L1271 (40.7875, 53.8779) -> (44.1633, 55.827)
  line L1272 (48.1421, 62.7184) -> (48.1421, 66.6164)
  line L1273 (49.3479, 62.7184) -> (52.7238, 60.7693)
  line L1274 (49.3479, 66.6164) -> (49.3479, 62.7184)
  line L1275 (52.7238, 68.5655) -> (49.3479, 66.6164)
  line L1276 (56.0996, 66.6164) -> (52.7238, 68.5655)
  line L1277 (52.7238, 60.7693) -> (56.0996, 62.7184)
  line L1278 (52.1208, 55.827) -> (52.1208, 59.725)
  line L1279 (52.1208, 59.725) -> (48.745, 61.6741)
  line L1280 (48.745, 61.6741) -> (45.3692, 59.725)
  line L1281 (45.3692, 59.725) -> (45.3692, 55.827)
  line L1282 (45.3692, 55.827) -> (48.745, 53.8779)
  line L1283 (48.745, 53.8779) -> (52.1208, 55.827)
  line L1284 (56.0996, 62.7184) -> (56.0996, 66.6164)
  line L1285 (57.3054, 62.7184) -> (60.6813, 60.7693)
  line L1286 (57.3054, 66.6164) -> (57.3054, 62.7184)
  line L1287 (60.6813, 68.5655) -> (57.3054, 66.6164)
  line L1288 (64.0571, 66.6164) -> (60.6813, 68.5655)
  line L1289 (60.6813, 60.7693) -> (64.0571, 62.7184)
  line L1290 (60.0783, 55.827) -> (60.0783, 59.725)
  line L1291 (60.0783, 59.725) -> (56.7025, 61.6741)
  line L1292 (56.7025, 61.6741) -> (53.3267, 59.725)
  line L1293 (53.3267, 59.725) -> (53.3267, 55.827)
  line L1294 (53.3267, 55.827) -> (56.7025, 53.8779)
  line L1295 (56.7025, 53.8779) -> (60.0783, 55.827)
  line L1296 (64.0571, 62.7184) -> (64.0571, 66.6164)
  line L1297 (65.2629, 62.7184) -> (68.6388, 60.7693)
  line L1298 (65.2629, 66.6164) -> (65.2629, 62.7184)
  line L1299 (68.6388, 68.5655) -> (65.2629, 66.6164)
  line L1300 (72.0146, 66.6164) -> (68.6388, 68.5655)
  line L1301 (68.6388, 60.7693) -> (72.0146, 62.7184)
  line L1302 (68.0358, 55.827) -> (68.0358, 59.725)
  line L1303 (68.0358, 59.725) -> (64.66, 61.6741)
  line L1304 (64.66, 61.6741) -> (61.2842, 59.725)
  line L1305 (61.2842, 59.725) -> (61.2842, 55.827)
  line L1306 (61.2842, 55.827) -> (64.66, 53.8779)
  line L1307 (64.66, 53.8779) -> (68.0358, 55.827)
  line L1308 (72.0146, 62.7184) -> (72.0146, 66.6164)
  line L1309 (73.2204, 62.7184) -> (76.5963, 60.7693)
  line L1310 (73.2204, 66.6164) -> (73.2204, 62.7184)
  line L1311 (76.5963, 68.5655) -> (73.2204, 66.6164)
  line L1312 (79.9721, 66.6164) -> (76.5963, 68.5655)
  line L1313 (76.5963, 60.7693) -> (79.9721, 62.7184)
  line L1314 (75.9933, 55.827) -> (75.9933, 59.725)
  line L1315 (75.9933, 59.725) -> (72.6175, 61.6741)
  line L1316 (72.6175, 61.6741) -> (69.2417, 59.725)
  line L1317 (69.2417, 59.725) -> (69.2417, 55.827)
  line L1318 (69.2417, 55.827) -> (72.6175, 53.8779)
  line L1319 (72.6175, 53.8779) -> (75.9933, 55.827)
  line L1320 (79.9721, 62.7184) -> (79.9721, 66.6164)
  line L1321 (81.1779, 62.7184) -> (84.5538, 60.7693)
  line L1322 (81.1779, 66.6164) -> (81.1779, 62.7184)
  line L1323 (84.5538, 68.5655) -> (81.1779, 66.6164)
  line L1324 (87.9296, 66.6164) -> (84.5538, 68.5655)
  line L1325 (84.5538, 60.7693) -> (87.9296, 62.7184)
  line L1326 (83.9508, 55.827) -> (83.9508, 59.725)
  line L1327 (83.9508, 59.725) -> (80.575, 61.6741)
  line L1328 (80.575, 61.6741) -> (77.1992, 59.725)
  line L1329 (77.1992, 59.725) -> (77.1992, 55.827)
  line L1330 (77.1992, 55.827) -> (80.575, 53.8779)
  line L1331 (80.575, 53.8779) -> (83.9508, 55.827)
  line L1332 (87.9296, 62.7184) -> (87.9296, 66.6164)
  line L1333 (1.6029, 76.6624) -> (4.9788, 74.7133)
  line L1334 (1.6029, 80.5604) -> (1.6029, 76.6624)
  line L1335 (4.9788, 82.5095) -> (1.6029, 80.5604)
  line L1336 (8.3546, 80.5604) -> (4.9788, 82.5095)
  line L1337 (4.9788, 74.7133) -> (8.3546, 76.6624)
  line L1338 (4.3758, 69.771) -> (4.3758, 73.669)
  line L1339 (4.3758, 73.669) -> (1, 75.6181)
  line L1340 (1, 75.6181) -> (-2.3758, 73.669)
  line L1341 (-2.3758, 73.669) -> (-2.3758, 69.771)
  line L1342 (-2.3758, 69.771) -> (1, 67.8219)
  line L1343 (1, 67.8219) -> (4.3758, 69.771)
  line L1344 (8.3546, 76.6624) -> (8.3546, 80.5604)
  line L1345 (9.5604, 76.6624) -> (12.9363, 74.7133)
  line L1346 (9.5604, 80.5604) -> (9.5604, 76.6624)
  line L1347 (12.9363, 82.5095) -> (9.5604, 80.5604)
  line L1348 (16.3121, 80.5604) -> (12.9363, 82.5095)
  line L1349 (12.9363, 74.7133) -> (16.3121, 76.6624)
  line L1350 (12.3333, 69.771) -> (12.3333, 73.669)
  line L1351 (12.3333, 73.669) -> (8.9575, 75.6181)
  line L1352 (8.9575, 75.6181) -> (5.5817, 73.669)
  line L1353 (5.5817, 73.669) -> (5.5817, 69.771)
  line L1354 (5.5817, 69.771) -> (8.9575, 67.8219)
  line L1355 (8.9575, 67.8219) -> (12.3333, 69.771)
  line L1356 (16.3121, 76.6624) -> (16.3121, 80.5604)
  line L1357 (17.5179, 76.6624) -> (20.8938, 74.7133)
  line L1358 (17.5179, 80.5604) -> (17.5179, 76.6624)
  line L1359 (20.8938, 82.5095) -> (17.5179, 80.5604)
  line L1360 (24.2696, 80.5604) -> (20.8938, 82.5095)
  line L1361 (20.8938, 74.7133) -> (24.2696, 76.6624)
  line L1362 (20.2908, 69.771) -> (20.2908, 73.669)
  line L1363 (20.2908, 73.669) -> (16.915, 75.6181)
  line L1364 (16.915, 75.6181) -> (13.5392, 73.669)
  line L1365 (13.5392, 73.669) -> (13.5392, 69.771)
  line L1366 (13.5392, 69.771) -> (16.915, 67.8219)
  line L1367 (16.915, 67.8219) -> (20.2908, 69.771)
  line L1368 (24.2696, 76.6624) -> (24.2696, 80.5604)
  line L1369 (25.4754, 76.6624) -> (28.8513, 74.7133)
  line L1370 (25.4754, 80.5604) -> (25.4754, 76.6624)
  line L1371 (28.8513, 82.5095) -> (25.4754, 80.5604)
  line L1372 (32.2271, 80.5604) -> (28.8513, 82.5095)
  line L1373 (28.8513, 74.7133) -> (32.2271, 76.6624)
  line L1374 (28.2483, 69.771) -> (28.2483, 73.669)
  line L1375 (28.2483, 73.669) -> (24.8725, 75.6181)
  line L1376 (24.8725, 75.6181) -> (21.4967, 73.669)
  line L1377 (21.4967, 73.669) -> (21.4967, 69.771)
  line L1378 (21.4967, 69.771) -> (24.8725, 67.8219)
  line L1379 (24.8725, 67.8219) -> (28.2483, 69.771)
  line L1380 (32.2271, 76.6624) -> (32.2271, 80.5604)
  line L1381 (33.4329, 76.6624) -> (36.8088, 74.7133)
  line L1382 (33.4329, 80.5604) -> (33.4329, 76.6624)
  line L1383 (36.8088, 82.5095) -> (33.4329, 80.5604)
  line L1384 (40.1846, 80.5604) -> (36.8088, 82.5095)
  line L1385 (36.8088, 74.7133) -> (40.1846, 76.6624)
  line L1386 (36.2058, 69.771) -> (36.2058, 73.669)
  line L1387 (36.2058, 73.669) -> (32.83, 75.6181)
  line L1388 (32.83, 75.6181) -> (29.4542, 73.669)
  line L1389 (29.4542, 73.669) -> (29.4542, 69.771)
  line L1390 (29.4542, 69.771) -> (32.83, 67.8219)
  line L1391 (32.83, 67.8219) -> (36.2058, 69.771)
  line L1392 (40.1846, 76.6624) -> (40.1846, 80.5604)
  line L1393 (41.3904, 76.6624) -> (44.7663, 74.7133)
  line L1394 (41.3904, 80.5604) -> (41.3904, 76.6624)
  line L1395 (44.7663, 82.5095) -> (41.3904, 80.5604)
  line L1396 (48.1421, 80.5604) -> (44.7663, 82.5095)
  line L1397 (44.7663, 74.7133) -> (48.1421, 76.6624)
  line L1398 (44.1633, 69.771) -> (44.1633, 73.669)
  line L1399 (44.1633, 73.669) -> (40.7875, 75.6181)
  line L1400 (40.7875, 75.6181) -> (37.4117, 73.669)
  line L1401 (37.4117, 73.669) -> (37.4117, 69.771)
  line L1402 (37.4117, 69.771) -> (40.7875, 67.8219)
  line L1403 (40.7875, 67.8219) -> (44.1633, 69.771)
  line L1404 (48.1421, 76.6624) -> (48.1421, 80.5604)
  line L1405 (49.3479, 76.6624) -> (52.7238, 74.7133)
  line L1406 (49.3479, 80.5604) -> (49.3479, 76.6624)
  line L1407 (52.7238, 82.5095) -> (49.3479, 80.5604)
  line L1408 (56.0996, 80.5604) -> (52.7238, 82.5095)
  line L1409 (52.7238, 74.7133) -> (56.0996, 76.6624)
  line L1410 (52.1208, 69.771) -> (52.1208, 73.669)
  line L1411 (52.1208, 73.669) -> (48.745, 75.6181)
  line L1412 (48.745, 75.6181) -> (45.3692, 73.669)
  line L1413 (45.3692, 73.669) -> (45.3692, 69.771)
  line L1414 (45.3692, 69.771) -> (48.745, 67.8219)
  line L1415 (48.745, 67.8219) -> (52.1208, 69.771)
  line L1416 (56.0996, 76.6624) -> (56.0996, 80.5604)
  line L1417 (57.3054, 76.6624) -> (60.6813, 74.7133)
  line L1418 (57.3054, 80.5604) -> (57.3054, 76.6624)
  line L1419 (60.6813, 82.5095) -> (57.3054, 80.5604)
  line L1420 (64.0571, 80.5604) -> (60.6813, 82.5095)
  line L1421 (60.6813, 74.7133) -> (64.0571, 76.6624)
  line L1422 (60.0783, 69.771) -> (60.0783, 73.669)
  line L1423 (60.0783, 73.669) -> (56.7025, 75.6181)
  line L1424 (56.7025, 75.6181) -> (53.3267, 73.669)
  line L1425 (53.3267, 73.669) -> (53.3267, 69.771)
  line L1426 (53.3267, 69.771) -> (56.7025, 67.8219)
  line L1427 (56.7025, 67.8219) -> (60.0783, 69.771)
  line L1428 (64.0571, 76.6624) -> (64.0571, 80.5604)
  line L1429 (65.2629, 76.6624) -> (68.6388, 74.7133)
  line L1430 (65.2629, 80.5604) -> (65.2629, 76.6624)
  line L1431 (68.6388, 82.5095) -> (65.2629, 80.5604)
  line L1432 (72.0146, 80.5604) -> (68.6388, 82.5095)
  line L1433 (68.6388, 74.7133) -> (72.0146, 76.6624)
  line L1434 (68.0358, 69.771) -> (68.0358, 73.669)
  line L1435 (68.0358, 73.669) -> (64.66, 75.6181)
  line L1436 (64.66, 75.6181) -> (61.2842, 73.669)
  line L1437 (61.2842, 73.669) -> (61.2842, 69.771)
  line L1438 (61.2842, 69.771) -> (64.66, 67.8219)
  line L1439 (64.66, 67.8219) -> (68.0358, 69.771)
  line L1440 (72.0146, 76.6624) -> (72.0146, 80.5604)
  line L1441 (73.2204, 76.6624) -> (76.5963, 74.7133)
  line L1442 (73.2204, 80.5604) -> (73.2204, 76.6624)
  line L1443 (76.5963, 82.5095) -> (73.2204, 80.5604)
  line L1444 (79.9721, 80.5604) -> (76.5963, 82.5095)
  line L1445 (76.5963, 74.7133) -> (79.9721, 76.6624)
  line L1446 (75.9933, 69.771) -> (75.9933, 73.669)
  line L1447 (75.9933, 73.669) -> (72.6175, 75.6181)
  line L1448 (72.6175, 75.6181) -> (69.2417, 73.669)
  line L1449 (69.2417, 73.669) -> (69.2417, 69.771)
  line L1450 (69.2417, 69.771) -> (72.6175, 67.8219)
  line L1451 (72.6175, 67.8219) -> (75.9933, 69.771)
  line L1452 (79.9721, 76.6624) -> (79.9721, 80.5604)
  line L1453 (81.1779, 76.6624) -> (84.5538, 74.7133)
  line L1454 (81.1779, 80.5604) -> (81.1779, 76.6624)
  line L1455 (84.5538, 82.5095) -> (81.1779, 80.5604)
  line L1456 (87.9296, 80.5604) -> (84.5538, 82.5095)
  line L1457 (84.5538, 74.7133) -> (87.9296, 76.6624)
  line L1458 (83.9508, 69.771) -> (83.9508, 73.669)
  line L1459 (83.9508, 73.669) -> (80.575, 75.6181)
  line L1460 (80.575, 75.6181) -> (77.1992, 73.669)
  line L1461 (77.1992, 73.669) -> (77.1992, 69.771)
  line L1462 (77.1992, 69.771) -> (80.575, 67.8219)
  line L1463 (80.575, 67.8219) -> (83.9508, 69.771)
  line L1464 (87.9296, 76.6624) -> (87.9296, 80.5604)
  point P0 (1, 2)
  dimension "d50" = 2
  dimension "d53" = 7.9575
  dimension "d54" = 7.8
  dimension "d56" = 1.2
  dimension "d60" = 7.9575
  dimension "d61" = 13.944
  dimension "d62" = 1.2
  constraint horizontal L0
  constraint vertical L1
  constraint horizontal L2
  constraint vertical L3
  constraint coincident L0.start L3.end
  constraint coincident P0 L1.end
  constraint midpoint L4 L10.end
  constraint midpoint L8 L11.end
  constraint horizontal L18
  constraint vertical L19
  constraint horizontal L20
  constraint vertical L21
  constraint vertical L9
  constraint midpoint L9 L22.start
  constraint perpendicular L9 L22
  constraint vertical L47
  constraint horizontal L48
  constraint midpoint L47.end L48
  measures "d50" distance of L0.end P0
  measures "d56" distance of L22.start L22.end
  measures "d62" distance of L12.end L47.end
extrude "Extrude7" add sketch "Top" along normal blind 2.5 separate body contours L5 L23 L26 L49 | A1 A2 A4 L23 L26 A7 L40 L41 L49 L55 L56 | A4 L23 L49 | A7 A10 L47 L49 | A4 A11 L44 L49 | A6 A10 L47 L49 | A7 A10 L47 L49 | L8 L25 A7 L49 L50 | L8 L20 L25 L41 | L6 A4 L24 L49 L51 | A4 A11 L44 L49 | A5 A11 L44 L49 | L6 L22 L24 L40 | A6 A10 L47 L49 | A6 L47 L49 | A2 A9 L46 L48 | L8 A2 L20 L48 L53 | A2 A9 L46 L56 L57 | A5 A11 L44 L49 | A5 L44 L49 | L6 L17 L22 L40 | A6 L47 L49 | A1 L18 A2 L21 L48 L55 L56 | A2 A9 L48 L56 L57 | A3 A9 L46 L48 | A3 A9 L46 L57 | A5 L44 L49 | L6 A1 L17 L48 L52 | A1 A8 L45 L55 | A1 A8 L45 L48 | A2 L21 L48 | A3 A9 L48 L57 | A3 L46 L48 | A3 L46 L48 L57 | A1 A8 L48 L55 | A0 A8 L45 L48 L55 | A0 A8 L45 L48 | L7 L18 L21 L48 | A3 L48 L57 | A1 L18 L48 | A8 L55 | A0 L45 L48 | A0 L45 L48 | A8 L48 L55 picked at (55.1052, -59.8026) picked at (15.6112, -57.7424) picked at (58.7824, -57.0477) picked at (57.5151, -58.4062) picked at (11.1052, -59.8026) picked at (13.683, -58.4059) picked at (57.683, -58.4059) picked at (57.7399, 56.76) picked at (56.8289, 56.8741) picked at (13.5151, -58.4062) picked at (55.1067, 59.8093) picked at (57.683, 58.4059) picked at (56.8667, 59.3796) picked at (11.1052, 59.8026) picked at (56.4416, 58.7134) picked at (13.683, 58.4059) picked at (13.5151, 58.4062) makes body 4
extrude "Extrude8" cut sketch "Top Hex" along normal blind 5 keep common part bodies 4